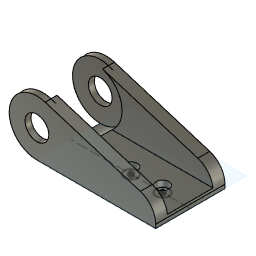
10x10_Drag_Chain_End (Autodesk Fusion 360 design; units mm, degrees)
Autodesk Fusion 360 part; units mm, degrees
sketch "Sketch1" plane through (0, 0, 0) normal (0, 1, 0) x (1, 0, 0)
  line L0 (0, 0) -> (30, 0)
  circle A0 centre (0, -7) radius 7
  circle A1 centre (0, -7) radius 3
  line L1 (30, 0) -> (30, -5)
  line L2 (30, -5) -> (2.0789, -13.6842)
  line L3 (30, -1.6) -> (4.4542, -1.6)
  dimension "d1" = 30
  dimension "d3" = 14
  dimension "d4" = 6
  dimension "d7" = 5
  dimension "d8" = 1.6
  constraint coincident L0.start origin
  constraint horizontal L0
  constraint tangent L0 A0
  constraint concentric A0 A1
  constraint vertical L1
  constraint coincident A0 L2.end
  constraint tangent A0 L2
  constraint vertical L0.start A0.centre
  constraint coincident L1 L3.start
  constraint coincident A0 L3.end
  constraint perpendicular L1 L3
  measures "d1" distance of L0.start L0.end
  measures "d3" diameter of A0
  measures "d4" diameter of A1
  measures "d7" distance of L0.end L1.end
  measures "d8" distance of L0 L3
ref_plane "WorkPlane1" through (0, 17.5, 0) normal (0, 1, 0) x (0, 0, 1)
sketch "Sketch2" plane through (0, 0, 0) normal (0, 1, 0) x (1, 0, 0)
sketch "Sketch3" plane through (0, 17.5, 0) normal (0, 1, 0) x (1, 0, 0)
  line L0 (30, -5) -> (2.0789, -13.6842)
  circle A0 centre (0, -7) radius 7
  circle A1 centre (0, -7) radius 3
  line L1 (30, -1.6) -> (4.4542, -1.6)
  line L2 (0, 0) -> (30, 0)
  line L3 (30, 0) -> (30, -5)
extrude "Extrude1" add sketch "Sketch1" along normal up to surface (17.5 mm away) contours L0 A0 L1 L3
extrude "Extrude2" add sketch "Sketch1" along normal blind 1.5 contours A0 | A0 L1 L2 L3
extrude "Extrude3" add sketch "Sketch1" along normal blind 3 contours A0 L1 L2 L3
extrude "Extrude4" add sketch "Sketch3" against normal blind 1.5 contours A0
extrude "Extrude5" add sketch "Sketch3" against normal blind 3 contours L0 A0 L1 L3
fillet "Fillet1" radius 5.5 2 edges at (30, 1.5, 5) (30, 16, 5)
sketch "Sketch4" plane through (0, 0, 0) normal (0, 0, -1) x (1, 0, 0)
  line L0 (0, -17.5) -> (30, -17.5)
  line L1 (30, -17.5) -> (30, 0)
  line L2 (30, 0) -> (0, 0)
  line L3 (0, 0) -> (0, -1.5)
  line L4 (0, -1.5) -> (0, -16)
  line L5 (0, -16) -> (0, -17.5)
  circle A0 centre (15, -8.75) radius 1.6
  circle A1 centre (23, -8.75) radius 1.6
  line L6 (30, -8.75) -> (0, -8.75) construction
  dimension "d24" = 3.2
  dimension "d25" = 3.2
  dimension "d27" = 8
  dimension "d30" = 15
  constraint midpoint L1 L6.start
  constraint midpoint L4 L6.end
  constraint coincident A0.centre L6
  constraint coincident A1.centre L6
  measures "d24" diameter of A0
  measures "d25" diameter of A1
  measures "d27" distance of A0.centre A1.centre
  measures "d30" distance of L4 A0.centre
extrude "Extrude6" cut sketch "Sketch4" against normal up to surface (1.6 mm away) contours A0 | A1
equation "d3 = CircleDiameter"
equation "d4 = SlotDiameter"
equation "SlotDiameter = 6 mm"
equation "CircleDiameter = 14 mm"
equation "d9 = Width"
equation "d12 = JointWallWidth"
equation "d14 = ThickWallWidth"
equation "d16 = -JointWallWidth"
equation "d18 = -ThickWallWidth"
equation "Width = 17.5 mm"
equation "JointWallWidth = 1.5 mm"
equation "ThickWallWidth = 3 mm"
equation "d25 = d24"
